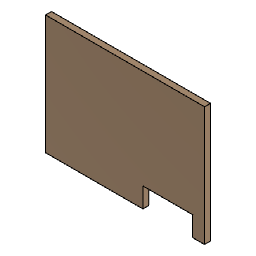
Connection box rear panel (Autodesk Fusion 360 design; units mm, degrees)
Autodesk Fusion 360 part; units mm, degrees
sketch "Sketch1" plane through (0, 0, 0) normal (0, 1, 0) x (1, 0, 0)
  line L0 (80, -60) -> (-80, -60)
  line L1 (-80, -60) -> (-80, 60)
  line L2 (-80, 60) -> (80, 60)
  line L3 (80, 60) -> (80, -60)
  line L4 (80, -60) -> (-80, 60) construction
  line L5 (-80, -60) -> (80, 60) construction
  line L6 (18, 60) -> (68, 60)
  line L7 (68, 60) -> (68, 40)
  line L8 (68, 40) -> (18, 40)
  line L9 (18, 40) -> (18, 60)
  dimension "d1" = 160
  dimension "d2" = 120
  dimension "d3" = 50
  dimension "d4" = 20
  dimension "d5" = 12
  constraint perpendicular L0 L1
  constraint parallel L0 L2
  constraint parallel L1 L3
  constraint horizontal L0
  constraint coincident L4 origin
  constraint coincident L5 origin
  constraint horizontal L6
  constraint vertical L7
  constraint horizontal L8
  constraint vertical L9
  constraint coincident L2 L6.start
  measures "d1" distance of L1.end L2.end
  measures "d2" distance of L0.end L1.end
  measures "d3" distance of L6.start L6.end
  measures "d4" distance of L6.start L8.end
  measures "d5" distance of L3 L7
extrude "Extrude1" add sketch "Sketch1" along normal blind 6 contours L0 L1 L2 L3 L7 L8 L9
named bodies: "Panel"
